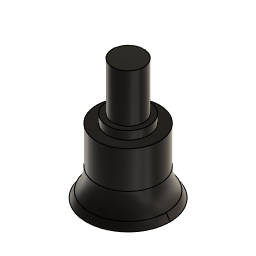
Knob (Autodesk Fusion 360 design; units mm, degrees)
Autodesk Fusion 360 part; units mm, degrees
sketch "Esquisse1" plane through (0, 0, 0) normal (0, 0, 1) x (1, 0, 0)
  circle A0 centre (0, 0) radius 20
  dimension "d1" = 40
  constraint coincident A0.centre origin
  measures "d1" diameter of A0
extrude "Extrusion1" add sketch "Esquisse1" along normal blind 1
sketch "Esquisse2" plane through (0, 0, 1) normal (0, 0, 1) x (-1, 0, 0)
  circle A0 centre (0, 0) radius 20
  circle A1 centre (0, 0) radius 15
  dimension "d4" = 30
  constraint coincident A0.centre A1.centre
  measures "d4" diameter of A1
extrude "Extrusion2" add sketch "Esquisse2" along normal blind 30 contours A1
fillet "Congé1" radius 17.5 1 faces at (18.203, -1.7388, 1)
sketch "Esquisse3" plane through (0, 0, 31) normal (0, 0, 1) x (-1, 0, 0)
  circle A0 centre (0, 0) radius 15
  circle A1 centre (0, 0) radius 10
  dimension "d9" = 20
  constraint coincident A0.centre A1.centre
  measures "d9" diameter of A1
extrude "Extrusion3" add sketch "Esquisse3" along normal blind 4 contours A1
sketch "Esquisse4" plane through (0, 0, 35) normal (0, 0, 1) x (-1, 0, 0)
  circle A0 centre (0, 0) radius 10
  circle A1 centre (0, 0) radius 7.5
  dimension "d12" = 15
  constraint coincident A0.centre A1.centre
  measures "d12" diameter of A1
extrude "Extrusion4" add sketch "Esquisse4" along normal blind 23 contours A1
